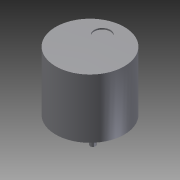
# Autodesk Inventor part: pidtech plus
Saved by Autodesk Inventor 2011 (Build 150239000, 239)
## iProperties
Created: 2012-04-20
Part Number: pidtech plus
Document SubType Name: Modeling
Designer: Marc
Density: 1 g/cm^3
pidTechPlusDia: 20.400 mm
pidTechPlusHeight: 17.600 mm
Author: Marc
Autodesk Inventor part; units mm, degrees
ref_plane "YZ Plane" through (0, 0, 0) normal (1, 0, 0) x (0, 1, 0)
ref_plane "XZ Plane" through (0, 0, 0) normal (0, 1, 0) x (-1, 0, 0)
ref_plane "XY Plane" through (0, 0, 0) normal (0, 0, 1) x (1, 0, 0)
sketch "Sketch1" plane through (0, 0, 0) normal (0, 0, 1) x (1, 0, 0)
  circle A0 centre (0, 0) radius 10.2
  dimension "pidTechPlusDia" = 20.4
  constraints: 1 centre point, 1 coincident
  measures "pidTechPlusDia" diameter of A0
extrude "Extrusion1" add sketch "Sketch1" along normal blind 17.6
sketch "Sketch2" plane through (0, 0, 17.6) normal (0, 0, 1) x (1, 0, 0)
  circle A0 centre (0, 0) radius 10.2 projected
  line L0 (0, 0) -> (-1.27, 0) construction
  line L1 (-1.27, 0) -> (-1.27, 4.93) construction
  line L2 (-1.27, 4.93) -> (0, 4.93) construction
  line L3 (0, 4.93) -> (0, 0) construction
  circle A1 centre (-1.27, 4.93) radius 2.415
  dimension "d3" = 1.27
  dimension "d4" = 4.93
  dimension "d5" = 4.83
  constraints: 8 end point, 2 parallel, 1 centre point, 1 coincident, 1 horizontal, 1 perpendicular
  measures "d3" distance of L1.end L2.end
  measures "d4" distance of L2.end L0.start
  measures "d5" diameter of A1
extrude "Extrusion2" cut sketch "Sketch2" against normal blind 0.4 contours A1
sketch "Sketch3" plane through (0, 0, 0) normal (0, 0, -1) x (-1, 0, 0)
  circle A0 centre (0, 0) radius 10.2 projected
  circle A1 centre (1.27, 4.93) radius 2.415 projected
  circle A2 centre (1.27, 4.93) radius 2.415 projected
  line L0 (0, 10.2) -> (0, -10.2) construction
  line L1 (-10.2, 0) -> (10.2, 0) construction
  circle A3 centre (4.24, 0) radius 0.785
  circle A4 centre (-3.38, 2.54) radius 0.785
  circle A5 centre (-3.38, -2.54) radius 0.785
  dimension "d8" = 4.24
  dimension "pinDia" = 1.57
  dimension "d10" = 7.62
  dimension "d11" = 5.08
  constraints: 4 end point, 4 point on circle, 3 centre point, 3 symmetric about line, 1 equal radius, 1 perpendicular, 1 point on line, 1 vertical, 1 other
  measures "d8" distance from line of L0 A3.centre
  measures "pinDia" diameter of A3
  measures "d10" horizontal distance of A3.centre A4.centre
  measures "d11" distance of A5.centre A4.centre
extrude "Extrusion3" add sketch "Sketch3" along normal blind 4.78 contours A3 | A4 | A5
body "Solid1"
